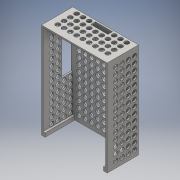
# Autodesk Inventor part: RaspPiCase
Saved by Autodesk Inventor 2016 (Build 200138000, 138)
## iProperties
Created: 2016-04-29
Part Number: RaspPiCase
Material: Generic
Document SubType Name: Modeling
Designer: mkepler
Density: 1 g/cm^3
Appearance: Default
Author: mkepler
Autodesk Inventor part; units mm, degrees
ref_plane "YZ Plane" through (0, 0, 0) normal (1, 0, 0) x (0, 1, 0)
ref_plane "XZ Plane" through (0, 0, 0) normal (0, 1, 0) x (-1, 0, 0)
ref_plane "XY Plane" through (0, 0, 0) normal (0, 0, 1) x (1, 0, 0)
sketch "Sketch1" plane through (0, 0, 0) normal (0, 1, 0) x (-1, 0, 0)
  line L0 (0, 0) -> (60, 0)
  line L1 (60, 0) -> (60, -90)
  line L2 (60, -90) -> (0, -90)
  line L3 (0, -90) -> (0, 0)
  circle A0 centre (6, -6) radius 2.15
  circle A1 centre (6, -12) radius 2.15
  circle A2 centre (12, -12) radius 2.15
  circle A3 centre (12, -6) radius 2.15
  line L4 (0, 0) -> (15, 0)
  line L5 (15, -28.7108) -> (16.2859, -28.7108)
  circle A4 centre (24, -6) radius 2.15
  circle A5 centre (24, -12) radius 2.15
  circle A6 centre (18, -12) radius 2.15
  circle A7 centre (18, -6) radius 2.15
  line L6 (0, 0) -> (27, 0)
  circle A8 centre (48, -6) radius 2.15
  circle A9 centre (48, -12) radius 2.15
  circle A10 centre (42, -12) radius 2.15
  circle A11 centre (42, -6) radius 2.15
  circle A12 centre (30, -6) radius 2.15
  circle A13 centre (36, -6) radius 2.15
  circle A14 centre (36, -12) radius 2.15
  circle A15 centre (30, -12) radius 2.15
  circle A16 centre (54, -6) radius 2.15
  circle A17 centre (54, -12) radius 2.15
  line L7 (60, 0) -> (60, -15)
  line L8 (60, 0) -> (60, -15)
  line L9 (60, -15) -> (56.15, -15)
  circle A18 centre (6, -24) radius 2.15
  circle A19 centre (6, -18) radius 2.15
  circle A20 centre (12, -18) radius 2.15
  circle A21 centre (12, -24) radius 2.15
  circle A22 centre (24, -24) radius 2.15
  circle A23 centre (18, -24) radius 2.15
  circle A24 centre (18, -18) radius 2.15
  circle A25 centre (24, -18) radius 2.15
  circle A26 centre (30, -24) radius 2.15
  circle A27 centre (30, -18) radius 2.15
  circle A28 centre (36, -24) radius 2.15
  circle A29 centre (36, -18) radius 2.15
  circle A30 centre (42, -24) radius 2.15
  circle A31 centre (42, -18) radius 2.15
  circle A32 centre (48, -18) radius 2.15
  circle A33 centre (48, -24) radius 2.15
  circle A34 centre (54, -24) radius 2.15
  circle A35 centre (54, -18) radius 2.15
  line L10 (60, 0) -> (60, -27)
  circle A36 centre (6, -42) radius 2.15
  circle A37 centre (12, -42) radius 2.15
  circle A38 centre (18, -42) radius 2.15
  circle A39 centre (24, -42) radius 2.15
  circle A40 centre (30, -42) radius 2.15
  circle A41 centre (36, -42) radius 2.15
  circle A42 centre (42, -42) radius 2.15
  circle A43 centre (48, -42) radius 2.15
  circle A44 centre (54, -42) radius 2.15
  circle A45 centre (54, -30) radius 2.15
  circle A46 centre (54, -36) radius 2.15
  circle A47 centre (48, -30) radius 2.15
  circle A48 centre (48, -36) radius 2.15
  circle A49 centre (42, -36) radius 2.15
  circle A50 centre (42, -30) radius 2.15
  circle A51 centre (36, -30) radius 2.15
  circle A52 centre (36, -36) radius 2.15
  circle A53 centre (30, -36) radius 2.15
  circle A54 centre (30, -30) radius 2.15
  circle A55 centre (24, -36) radius 2.15
  circle A56 centre (24, -30) radius 2.15
  circle A57 centre (18, -30) radius 2.15
  circle A58 centre (18, -36) radius 2.15
  circle A59 centre (12, -36) radius 2.15
  circle A60 centre (12, -30) radius 2.15
  circle A61 centre (6, -30) radius 2.15
  circle A62 centre (6, -36) radius 2.15
  line L11 (60, 0) -> (60, -45)
  line L12 (60, -45) -> (48.8128, -45)
  circle A63 centre (6, -84) radius 2.15
  circle A64 centre (6, -78) radius 2.15
  circle A65 centre (12, -78) radius 2.15
  circle A66 centre (12, -84) radius 2.15
  line L13 (15, -61.2892) -> (16.2859, -61.2892)
  circle A67 centre (24, -84) radius 2.15
  circle A68 centre (18, -84) radius 2.15
  circle A69 centre (18, -78) radius 2.15
  circle A70 centre (24, -78) radius 2.15
  circle A71 centre (30, -84) radius 2.15
  circle A72 centre (30, -78) radius 2.15
  circle A73 centre (36, -84) radius 2.15
  circle A74 centre (36, -78) radius 2.15
  circle A75 centre (42, -84) radius 2.15
  circle A76 centre (42, -78) radius 2.15
  circle A77 centre (48, -78) radius 2.15
  circle A78 centre (48, -84) radius 2.15
  circle A79 centre (54, -84) radius 2.15
  circle A80 centre (54, -78) radius 2.15
  line L14 (60, -75) -> (56.15, -75)
  circle A81 centre (54, -66) radius 2.15
  circle A82 centre (54, -72) radius 2.15
  circle A83 centre (48, -66) radius 2.15
  circle A84 centre (48, -72) radius 2.15
  circle A85 centre (42, -72) radius 2.15
  circle A86 centre (42, -66) radius 2.15
  circle A87 centre (36, -66) radius 2.15
  circle A88 centre (36, -72) radius 2.15
  circle A89 centre (30, -72) radius 2.15
  circle A90 centre (30, -66) radius 2.15
  circle A91 centre (24, -72) radius 2.15
  circle A92 centre (24, -66) radius 2.15
  circle A93 centre (18, -66) radius 2.15
  circle A94 centre (18, -72) radius 2.15
  circle A95 centre (12, -72) radius 2.15
  circle A96 centre (12, -66) radius 2.15
  circle A97 centre (6, -66) radius 2.15
  circle A98 centre (6, -72) radius 2.15
  circle A99 centre (54, -48) radius 2.15
  circle A100 centre (54, -54) radius 2.15
  circle A101 centre (54, -60) radius 2.15
  circle A102 centre (48, -60) radius 2.15
  circle A103 centre (48, -54) radius 2.15
  circle A104 centre (48, -48) radius 2.15
  circle A105 centre (42, -48) radius 2.15
  circle A106 centre (42, -54) radius 2.15
  circle A107 centre (42, -60) radius 2.15
  circle A108 centre (36, -60) radius 2.15
  circle A109 centre (36, -54) radius 2.15
  circle A110 centre (36, -48) radius 2.15
  circle A111 centre (30, -48) radius 2.15
  circle A112 centre (30, -54) radius 2.15
  circle A113 centre (30, -60) radius 2.15
  circle A114 centre (24, -60) radius 2.15
  circle A115 centre (24, -54) radius 2.15
  circle A116 centre (24, -48) radius 2.15
  circle A117 centre (18, -48) radius 2.15
  circle A118 centre (18, -54) radius 2.15
  circle A119 centre (18, -60) radius 2.15
  circle A120 centre (12, -60) radius 2.15
  circle A121 centre (12, -54) radius 2.15
  circle A122 centre (12, -48) radius 2.15
  circle A123 centre (6, -54) radius 2.15
  circle A124 centre (6, -48) radius 2.15
  circle A125 centre (6, -60) radius 2.15
  dimension "d0" = 60
  dimension "d1" = 4.3
  dimension "d2" = 6
  dimension "d3" = 6
  dimension "d4" = 4.3
  dimension "d5" = 6
  dimension "d6" = 90
  dimension "d7" = 4.3
  dimension "d8" = 6
  dimension "d9" = 4.3
  dimension "d10" = 15
  dimension "d12" = 27
  dimension "d13" = 4.3
  dimension "d14" = 4.3
  dimension "d15" = 6
  dimension "d16" = 6
  dimension "d17" = 15
  dimension "d18" = 27
  dimension "d19" = 45
  constraints: 126 centre point, 85 symmetric about line, 30 end point, 4 point on line, 2 horizontal, 2 parallel, 2 perpendicular, 1 collinear, 1 midpoint, 81 other
  measures "d0" distance of L1.end L2.end
  measures "d1" diameter of A0
  measures "d2" distance from line of L0 A0.centre
  measures "d3" distance from line of L3 A0.centre
  measures "d4" diameter of A1
  measures "d5" distance of A1.centre A0.centre
  measures "d6" distance of L0.end L1.end
  measures "d7" diameter of A2
  measures "d8" distance of A1.centre A2.centre
  measures "d9" diameter of A3
  measures "d10" distance of L0.start L4.end
  measures "d12" distance of L0.start L6.end
  measures "d13" diameter of A16
  measures "d14" diameter of A17
  measures "d15" distance of A8.centre A16.centre
  measures "d16" distance of A9.centre A17.centre
  measures "d17" distance of L0.end L7.end
  measures "d18" distance of L0.end L10.end
  measures "d19" distance of L0.end L11.end
extrude "Extrusion1" add sketch "Sketch1" along normal blind 1.5
sketch "Sketch3" plane through (0, 0, 0) normal (1, 0, 0) x (0, 0, -1)
  line L0 (0, 1.5) -> (90, 1.5) projected
  line L1 (0, 1.5) -> (90, 1.5)
  line L2 (90, 1.5) -> (90, -28.5)
  line L3 (90, -28.5) -> (0, -28.5)
  line L4 (0, -28.5) -> (0, 1.5)
  point P0 (0, 0)
  dimension "d25" = 90
  dimension "d26" = 30
  constraints: 8 end point, 2 parallel, 1 horizontal, 1 perpendicular
  measures "d25" distance of L2.end L3.end
  measures "d26" distance of L1.end L2.end
extrude "Extrusion3" add sketch "Sketch3" along normal blind 1.5
sketch "Sketch5" plane through (-60, 0, -90) normal (-1, 0, 0) x (0, 0, 1)
  line L0 (90, -28.5) -> (90, 0) projected
  line L1 (90, 1.5) -> (0, 1.5)
  line L2 (0, 1.5) -> (0, -28.5)
  line L3 (0, -28.5) -> (90, -28.5)
  line L4 (90, -28.5) -> (90, 1.5)
  dimension "d31" = 90
  dimension "d32" = 30
  constraints: 8 end point, 2 parallel, 1 horizontal, 1 perpendicular
  measures "d31" distance of L3.end L2.end
  measures "d32" distance of L2.end L1.end
extrude "Extrusion5" add sketch "Sketch5" along normal blind 1.5
sketch "Sketch8" plane through (0, 1.5, 0) normal (0, 1, 0) x (1, 0, 0)
  line L0 (-61.5, 0) -> (-61.5, 90) projected
  line L1 (-61.5, 0) -> (1.5, 0)
  line L2 (1.5, 0) -> (1.5, -1.5)
  line L3 (1.5, -1.5) -> (-61.5, -1.5)
  line L4 (-61.5, -1.5) -> (-61.5, 0)
  point P0 (0, 0)
  dimension "d40" = 63
  dimension "d41" = 1.5
  constraints: 8 end point, 2 parallel, 1 horizontal, 1 perpendicular
  measures "d40" distance of L2.end L3.end
  measures "d41" distance of L1.end L2.end
extrude "Extrusion7" add sketch "Sketch8" against normal blind 30
sketch "Sketch9" plane through (-61.5, 0, -90) normal (-1, 0, 0) x (0, 0, 1)
  circle A0 centre (84, -2.3) radius 2.15
  line L0 (91.5, 1.5) -> (91.5, -28.5) projected
  circle A1 centre (84, -8.3) radius 2.15
  line L1 (84, -2.3) -> (84, -8.3)
  line L2 (91.5, 1.5) -> (91.5, -28.5) projected
  line L3 (84, -8.3) -> (84, -11.3)
  line L4 (84, -11.3) -> (91.5, -11.3)
  circle A2 centre (84, -20.3) radius 2.15
  circle A3 centre (84, -14.3) radius 2.15
  line L5 (84, -20.3) -> (84, -14.3)
  line L6 (84, -14.3) -> (84, -11.3)
  line L7 (84, -2.3) -> (81, -2.3)
  line L8 (81, -2.3) -> (81, -28.5)
  circle A4 centre (78, -2.3) radius 2.15
  circle A5 centre (78, -8.3) radius 2.15
  line L9 (78, -2.3) -> (78, -8.3)
  line L10 (78, -8.3) -> (78, -11.3)
  line L11 (78, -11.3) -> (70.5, -11.3)
  circle A6 centre (78, -20.3) radius 2.15
  circle A7 centre (78, -14.3) radius 2.15
  line L12 (78, -20.3) -> (78, -14.3)
  line L13 (78, -14.3) -> (78, -11.3)
  line L14 (78, -2.3) -> (81, -2.3)
  line L15 (78, -20.3) -> (75, -20.3)
  line L16 (75, -20.3) -> (75, -8.9833)
  circle A8 centre (66, -2.3) radius 2.15
  circle A9 centre (66, -8.3) radius 2.15
  line L17 (66, -11.3) -> (58.5, -11.3)
  circle A10 centre (66, -20.3) radius 2.15
  circle A11 centre (66, -14.3) radius 2.15
  line L18 (69, -2.3) -> (69, -28.5)
  circle A12 centre (72, -2.3) radius 2.15
  line L19 (72, -11.3) -> (79.5, -11.3)
  circle A13 centre (72, -8.3) radius 2.15
  circle A14 centre (72, -14.3) radius 2.15
  circle A15 centre (72, -20.3) radius 2.15
  line L20 (72, -20.3) -> (75, -20.3)
  line L21 (66, -20.3) -> (63, -20.3)
  line L22 (63, -20.3) -> (63, -15.4)
  circle A16 centre (42, -2.3) radius 2.15
  circle A17 centre (42, -8.3) radius 2.15
  line L23 (42, -2.3) -> (42, -8.3)
  line L24 (42, -8.3) -> (42, -11.3)
  circle A18 centre (42, -20.3) radius 2.15
  circle A19 centre (42, -14.3) radius 2.15
  line L25 (42, -20.3) -> (42, -14.3)
  line L26 (42, -14.3) -> (42, -11.3)
  line L27 (42, -2.3) -> (45, -2.3)
  line L28 (48, -2.3) -> (48, -8.3)
  circle A20 centre (48, -2.3) radius 2.15
  line L29 (48, -2.3) -> (45, -2.3)
  line L30 (48, -11.3) -> (55.5, -11.3)
  line L31 (48, -8.3) -> (48, -11.3)
  circle A21 centre (48, -8.3) radius 2.15
  line L32 (48, -14.3) -> (48, -11.3)
  circle A22 centre (48, -14.3) radius 2.15
  line L33 (48, -20.3) -> (48, -14.3)
  circle A23 centre (48, -20.3) radius 2.15
  line L34 (48, -20.3) -> (51, -20.3)
  line L35 (51, -20.3) -> (51, -8.9833)
  circle A24 centre (60, -2.3) radius 2.15
  circle A25 centre (54, -14.3) radius 2.15
  circle A26 centre (60, -14.3) radius 2.15
  line L36 (54, -20.3) -> (51, -20.3)
  circle A27 centre (60, -20.3) radius 2.15
  circle A28 centre (54, -20.3) radius 2.15
  circle A29 centre (54, -8.3) radius 2.15
  circle A30 centre (60, -8.3) radius 2.15
  line L37 (54, -11.3) -> (46.5, -11.3)
  circle A31 centre (54, -2.3) radius 2.15
  line L38 (42, -20.3) -> (39, -20.3)
  line L39 (39, -20.3) -> (39, -14.6416)
  circle A32 centre (12, -2.3) radius 2.15
  circle A33 centre (6, -14.3) radius 2.15
  circle A34 centre (12, -14.3) radius 2.15
  circle A35 centre (12, -20.3) radius 2.15
  circle A36 centre (6, -20.3) radius 2.15
  circle A37 centre (6, -8.3) radius 2.15
  circle A38 centre (12, -8.3) radius 2.15
  circle A39 centre (6, -2.3) radius 2.15
  line L40 (12, -20.3) -> (15, -20.3)
  line L41 (15, -20.3) -> (15, -15.4)
  circle A40 centre (18, -20.3) radius 2.15
  circle A41 centre (24, -20.3) radius 2.15
  line L42 (30, -20.3) -> (27, -20.3)
  line L43 (30, -20.3) -> (30, -14.3)
  line L44 (30, -11.3) -> (22.5, -11.3)
  line L45 (30, -14.3) -> (30, -11.3)
  circle A42 centre (30, -20.3) radius 2.15
  line L46 (24, -11.3) -> (31.5, -11.3)
  circle A43 centre (30, -14.3) radius 2.15
  line L47 (30, -8.3) -> (30, -11.3)
  line L48 (36, -20.3) -> (36, -14.3)
  circle A44 centre (36, -20.3) radius 2.15
  circle A45 centre (36, -2.3) radius 2.15
  line L49 (24, -20.3) -> (27, -20.3)
  line L50 (30, -2.3) -> (30, -8.3)
  line L51 (30, -2.3) -> (33, -2.3)
  circle A46 centre (30, -2.3) radius 2.15
  circle A47 centre (30, -8.3) radius 2.15
  circle A48 centre (36, -8.3) radius 2.15
  line L52 (36, -2.3) -> (36, -8.3)
  line L53 (36, -8.3) -> (36, -11.3)
  circle A49 centre (36, -14.3) radius 2.15
  line L54 (36, -14.3) -> (36, -11.3)
  line L55 (36, -2.3) -> (33, -2.3)
  circle A50 centre (24, -14.3) radius 2.15
  circle A51 centre (24, -8.3) radius 2.15
  circle A52 centre (24, -2.3) radius 2.15
  circle A53 centre (18, -8.3) radius 2.15
  circle A54 centre (18, -2.3) radius 2.15
  circle A55 centre (18, -14.3) radius 2.15
  line L56 (36, -20.3) -> (39, -20.3)
  point P0 (90, 0)
  point P1 (57, -2.3)
  point P2 (60, -11.3)
  point P3 (18, -11.3)
  point P4 (21, -2.3)
  dimension "d44" = 4.3
  dimension "d46" = 7.5
  dimension "d47" = 4.3
  dimension "d48" = 6
  dimension "d49" = 3
  dimension "d50" = 3
  dimension "d51" = 3
  dimension "d52" = 3
  dimension "d53" = 3
  constraints: 110 end point, 83 symmetric about line, 56 centre point, 13 point on line, 4 horizontal, 4 perpendicular, 1 parallel, 1 vertical, 54 other
  measures "d44" diameter of A0
  measures "d46" distance from line of L0 L1.start
  measures "d47" diameter of A1
  measures "d48" distance of L1.start L1.end
  measures "d49" distance of L1.end L3.end
  measures "d50" distance of L1.start L7.end
  measures "d51" distance of L12.start L15.end
  measures "d52" distance of L21.start L21.end
  measures "d53" distance of L25.start L38.end
hole "Hole1" at (-61.5, -20.3, -6) at (-61.5, -20.3, -12) at (-61.5, -20.3, -18) at (-61.5, -20.3, -24) at (-61.5, -20.3, -30) at (-61.5, -20.3, -36) at (-61.5, -20.3, -42) at (-61.5, -20.3, -48) at (-61.5, -20.3, -54) at (-61.5, -20.3, -60) at (-61.5, -20.3, -66) at (-61.5, -20.3, -72) at (-61.5, -20.3, -78) at (-61.5, -20.3, -84) at (-61.5, -14.3, -84) at (-61.5, -14.3, -78) at (-61.5, -14.3, -72) at (-61.5, -14.3, -66) at (-61.5, -14.3, -60) at (-61.5, -14.3, -54) at (-61.5, -14.3, -48) at (-61.5, -14.3, -42) at (-61.5, -14.3, -36) at (-61.5, -14.3, -30) at (-61.5, -14.3, -24) at (-61.5, -14.3, -18) at (-61.5, -14.3, -12) at (-61.5, -14.3, -6) at (-61.5, -8.3, -6) at (-61.5, -8.3, -12) at (-61.5, -8.3, -18) at (-61.5, -8.3, -24) at (-61.5, -8.3, -30) at (-61.5, -8.3, -36) at (-61.5, -8.3, -42) at (-61.5, -8.3, -48) at (-61.5, -8.3, -54) at (-61.5, -8.3, -60) at (-61.5, -8.3, -66) at (-61.5, -8.3, -72) at (-61.5, -8.3, -78) at (-61.5, -8.3, -84) at (-61.5, -2.3, -84) at (-61.5, -2.3, -78) at (-61.5, -2.3, -72) at (-61.5, -2.3, -66) at (-61.5, -2.3, -60) at (-61.5, -2.3, -54) at (-61.5, -2.3, -48) at (-61.5, -2.3, -42) direction (1, 0, 0) diameter 4.3 end through all and at (-61.5, -2.3, -36) (-61.5, -2.3, -30) (-61.5, -2.3, -24) (-61.5, -2.3, -18) (-61.5, -2.3, -12) (-61.5, -2.3, -6)
sketch "Sketch10" plane through (-61.5, 1.5, 1.5) normal (0, 0, 1) x (1, 0, 0)
  circle A0 centre (7.5, -3.8) radius 2.15
  line L0 (63, 0) -> (0, 0) projected
  line L1 (0, 0) -> (0, -30) projected
  circle A1 centre (13.5, -3.8) radius 2.15
  circle A2 centre (7.5, -9.8) radius 2.15
  circle A3 centre (13.5, -9.8) radius 2.15
  line L2 (7.5, -9.8) -> (7.5, -12.8)
  line L3 (7.5, -12.8) -> (8.9551, -12.8)
  circle A4 centre (7.5, -21.8) radius 2.15
  circle A5 centre (13.5, -21.8) radius 2.15
  circle A6 centre (7.5, -15.8) radius 2.15
  circle A7 centre (13.5, -15.8) radius 2.15
  line L4 (7.5, -15.8) -> (7.5, -12.8)
  line L5 (13.5, -3.8) -> (16.5, -3.8)
  line L6 (16.5, -3.8) -> (16.5, -8.3155)
  circle A8 centre (25.5, -3.8) radius 2.15
  circle A9 centre (19.5, -3.8) radius 2.15
  circle A10 centre (25.5, -9.8) radius 2.15
  circle A11 centre (19.5, -9.8) radius 2.15
  line L7 (25.5, -9.8) -> (25.5, -12.8)
  line L8 (25.5, -12.8) -> (24.0449, -12.8)
  circle A12 centre (25.5, -21.8) radius 2.15
  circle A13 centre (19.5, -21.8) radius 2.15
  circle A14 centre (25.5, -15.8) radius 2.15
  circle A15 centre (19.5, -15.8) radius 2.15
  line L9 (25.5, -15.8) -> (25.5, -12.8)
  line L10 (19.5, -3.8) -> (16.5, -3.8)
  line L11 (25.5, -3.8) -> (28.5, -3.8)
  line L12 (28.5, -3.8) -> (28.5, -7.65)
  circle A16 centre (49.5, -3.8) radius 2.15
  circle A17 centre (43.5, -3.8) radius 2.15
  circle A18 centre (49.5, -9.8) radius 2.15
  circle A19 centre (43.5, -9.8) radius 2.15
  line L13 (49.5, -9.8) -> (49.5, -12.8)
  line L14 (49.5, -12.8) -> (48.0449, -12.8)
  circle A20 centre (49.5, -21.8) radius 2.15
  circle A21 centre (43.5, -21.8) radius 2.15
  circle A22 centre (49.5, -15.8) radius 2.15
  circle A23 centre (43.5, -15.8) radius 2.15
  line L15 (49.5, -15.8) -> (49.5, -12.8)
  line L16 (43.5, -3.8) -> (40.5, -3.8)
  line L17 (40.5, -3.8) -> (40.5, -8.3155)
  line L18 (31.5, -12.8) -> (32.9551, -12.8)
  line L19 (31.5, -15.8) -> (31.5, -12.8)
  circle A24 centre (37.5, -15.8) radius 2.15
  circle A25 centre (37.5, -21.8) radius 2.15
  circle A26 centre (31.5, -21.8) radius 2.15
  circle A27 centre (31.5, -15.8) radius 2.15
  line L20 (31.5, -9.8) -> (31.5, -12.8)
  circle A28 centre (31.5, -9.8) radius 2.15
  circle A29 centre (37.5, -9.8) radius 2.15
  circle A30 centre (31.5, -3.8) radius 2.15
  line L21 (37.5, -3.8) -> (40.5, -3.8)
  circle A31 centre (37.5, -3.8) radius 2.15
  line L22 (49.5, -3.8) -> (52.5, -3.8)
  line L23 (52.5, -3.8) -> (52.5, -9.251)
  circle A32 centre (55.5, -3.8) radius 2.15
  circle A33 centre (55.5, -9.8) radius 2.15
  line L24 (55.5, -9.8) -> (55.5, -12.8)
  line L25 (55.5, -12.8) -> (56.9551, -12.8)
  circle A34 centre (55.5, -21.8) radius 2.15
  circle A35 centre (55.5, -15.8) radius 2.15
  line L26 (55.5, -15.8) -> (55.5, -12.8)
  line L27 (55.5, -3.8) -> (52.5, -3.8)
  point P0 (61.5, -1.5)
  dimension "d61" = 4.3
  dimension "d62" = 3.8
  dimension "d63" = 7.5
  dimension "d64" = 4.3
  dimension "d65" = 6
  dimension "d66" = 4.3
  dimension "d67" = 6
  dimension "d68" = 4.3
  dimension "d69" = 3
  dimension "d70" = 3
  dimension "d71" = 3
  dimension "d72" = 3
  constraints: 52 end point, 42 symmetric about line, 36 centre point, 4 horizontal, 3 perpendicular, 1 vertical, 32 other
  measures "d61" diameter of A0
  measures "d62" distance from line of L0 A0.centre
  measures "d63" distance from line of L1 A0.centre
  measures "d64" diameter of A1
  measures "d65" distance of L5.start A0.centre
  measures "d66" diameter of A2
  measures "d67" distance of L2.start A0.centre
  measures "d68" diameter of A3
  measures "d69" distance of L2.start L2.end
  measures "d70" distance of L5.start L5.end
  measures "d71" distance of L11.start L11.end
  measures "d72" distance of L22.start L22.end
hole "Hole2" at (-54, -20.3, 1.5) at (-48, -20.3, 1.5) at (-42, -20.3, 1.5) at (-36, -20.3, 1.5) at (-54, -14.3, 1.5) at (-48, -14.3, 1.5) at (-54, -8.3, 1.5) at (-54, -2.3, 1.5) at (-48, -8.3, 1.5) at (-48, -2.3, 1.5) at (-42, -2.3, 1.5) at (-42, -8.3, 1.5) at (-42, -14.3, 1.5) at (-36, -14.3, 1.5) at (-36, -8.3, 1.5) at (-36, -2.3, 1.5) at (-30, -2.3, 1.5) at (-30, -8.3, 1.5) at (-30, -14.3, 1.5) at (-30, -20.3, 1.5) at (-24, -20.3, 1.5) at (-24, -14.3, 1.5) at (-24, -8.3, 1.5) at (-24, -2.3, 1.5) at (-18, -20.3, 1.5) at (-18, -14.3, 1.5) at (-18, -8.3, 1.5) at (-18, -2.3, 1.5) at (-12, -20.3, 1.5) at (-6, -20.3, 1.5) at (-12, -14.3, 1.5) at (-6, -14.3, 1.5) at (-6, -8.3, 1.5) at (-12, -8.3, 1.5) at (-12, -2.3, 1.5) at (-6, -2.3, 1.5) direction (0, 0, -1) diameter 4.3 end through all
sketch "Sketch11" plane through (-61.5, 1.5, 1.5) normal (0, 0, 1) x (1, 0, 0)
  line L0 (1.5, -1.5) -> (61.5, -1.5) projected
  line L1 (39.65, -1.5) -> (23.1579, -1.5)
  line L2 (23.1579, -1.5) -> (23.1579, -5.95)
  line L3 (23.1579, -5.95) -> (39.65, -5.95)
  line L4 (39.65, -5.95) -> (39.65, -1.5)
  constraints: 8 end point, 2 parallel, 1 horizontal, 1 perpendicular, 1 point on line
extrude "Extrusion8" cut sketch "Sketch11" against normal blind 30
sketch "Sketch12" plane through (-60, 0, -90) normal (1, 0, 0) x (0, 0, -1)
  line L0 (0, 0) -> (-90, 0) projected
  line L1 (0, -28.5) -> (-90, -28.5) projected
  line L2 (0, 0) -> (-3.7, 0)
  line L3 (-3.7, 0) -> (-3.7, -28.5)
  line L4 (-3.7, -28.5) -> (0, -28.5)
  line L5 (0, -28.5) -> (0, 0)
  dimension "d82" = 3.7
  constraints: 8 end point, 2 parallel, 1 horizontal, 1 perpendicular, 1 point on line
  measures "d82" distance of L4.end L3.end
extrude "Extrusion9" add sketch "Sketch12" along normal blind 2
sketch "Sketch13" plane through (0, 0, 0) normal (-1, 0, 0) x (0, 0, 1)
  line L0 (-90, -28.5) -> (0, -28.5) projected
  line L1 (-90, 0) -> (-86.3, 0)
  line L2 (-86.3, 0) -> (-86.3, -28.5)
  line L3 (-86.3, -28.5) -> (-90, -28.5)
  line L4 (-90, -28.5) -> (-90, 0)
  point P0 (0, 0)
  dimension "d85" = 3.7
  constraints: 8 end point, 2 parallel, 1 horizontal, 1 perpendicular, 1 point on line
  measures "d85" distance of L2.end L3.end
extrude "Extrusion10" add sketch "Sketch13" along normal blind 2
sketch "Sketch14" plane through (0, 0, 0) normal (-1, 0, 0) x (0, 0, 1)
  point P0 (0, 0)
sketch "Sketch15" plane through (-61.5, 0, -90) normal (-1, 0, 0) x (0, 0, 1)
  line L0 (80.65, 0) -> (75.15, 0)
  line L1 (3.7, 0) -> (90, 0) projected
  line L2 (75.15, -10.5402) -> (80.65, -10.5402)
  line L3 (80.65, -10.5402) -> (80.65, 0)
  line L4 (74.8403, 0) -> (69.3403, 0)
  line L5 (69.3403, -10.5402) -> (75.15, -10.5402)
  line L6 (75.15, 0) -> (54.15, 0)
  line L7 (54.15, 0) -> (64.15, 0)
  line L8 (68.15, 0) -> (63.85, 0) projected
  line L9 (69.3403, -10.5402) -> (39.1728, -10.5402)
  line L10 (80.65, 0) -> (80.65, -10.5402)
  line L11 (80.65, 0) -> (39.1728, 0)
  line L12 (39.1728, 0) -> (39.1728, -10.5402)
  point P0 (86.15, 0)
  dimension "d93" = 11
  dimension "d95" = 5.5
  constraints: 22 end point, 2 point on line, 1 horizontal, 1 perpendicular, 6 other
  measures "d93" distance of point (86.15, 0) L0.end
  measures "d95" distance of L2.start L2.end
extrude "Extrusion11" cut sketch "Sketch15" against normal blind 2
sketch "Sketch16" plane through (0, 0, 0) normal (0, -1, 0) x (1, 0, 0)
  point P0 (0, 0)
body "Solid1"
